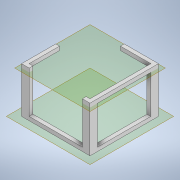
# Autodesk Inventor part: mousecap
Saved by Autodesk Inventor 2022 (Build 260153000, 153)
## iProperties
Created: 2022-02-16
Part Number: mousecap
Material: Generic
Document SubType Name: Modeling
Designer: Cornell
Density: 1 g/cm^3
Appearance: Default
Author: Cornell
Autodesk Inventor part; units mm, degrees
ref_plane "YZ Plane" through (0, 0, 0) normal (1, 0, 0) x (0, 1, 0)
ref_plane "XZ Plane" through (0, 0, 0) normal (0, 1, 0) x (-1, 0, 0)
ref_plane "XY Plane" through (0, 0, 0) normal (0, 0, 1) x (1, 0, 0)
sketch "Sketch1" plane through (0, 0, 0) normal (0, 1, 0) x (-1, 0, 0)
  line L0 (-9, -9) -> (-9, 9)
  line L1 (-9, 9) -> (9, 9)
  line L2 (-8, -8) -> (-8, 8)
  line L3 (-8, 8) -> (8, 8)
  line L4 (0, -8) -> (0, -9)
  line L5 (0, -9) -> (-1, -9)
  line L6 (-8, -8) -> (0, -8)
  line L7 (-9, -9) -> (0, -9)
  line L8 (9, 0) -> (9, 9)
  line L9 (8, 8) -> (8, 1)
  line L10 (9, 0) -> (8, 0)
  line L11 (8, 0) -> (8, 1.1953)
  line L12 (8, 8) -> (8, 9)
  line L13 (-8, 8) -> (-8, 9)
  line L14 (9, 9) -> (8, 9)
  line L15 (-8, 9) -> (-9, 9)
  line L16 (8, 8) -> (7, 8)
  line L17 (7, 8) -> (7, 9)
  line L18 (-8, 8) -> (-7, 8)
  line L19 (-7, 9) -> (-8, 9)
  line L20 (-8, 8) -> (-7, 8)
  line L21 (-7, 8) -> (-7, 9)
  point P0 (0, 0)
  point P1 (0, 11.1675)
  dimension "d4" = 18
  dimension "d5" = 18
  dimension "d10" = 16
  dimension "d11" = 16
  dimension "d33" = 1
  dimension "d62" = 1
  dimension "d63" = 1
  constraints: 44 end point, 8 point on line, 5 perpendicular, 4 collinear, 2 horizontal, 1 vertical
  measures "d4" distance of L0.start L0.end
  measures "d5" distance of L0.end L1.end
  measures "d10" distance of L2.start L2.end
  measures "d11" distance of L2.end L3.end
  measures "d33" distance of L4.end L5.end
  measures "d62" distance of L3.end L16.end
  measures "d63" distance of L2.end L18.end
extrude "Extrusion1" add sketch "Sketch1" against normal blind 1 contours L0 L1 L13 L2 L6 L4 L5 L7 | L1 L21 L3 L13 | L1 L12 L3 L17 | L1 L8 L10 L11 L9 L12
ref_plane "Work Plane1" through (0, -12, 0) normal (0, -1, 0) x (1, 0, 0)
ref_plane "Work Plane6" through (0, -1, 0) normal (0, -1, 0) x (1, 0, 0)
sketch "Sketch11" plane through (0, -1, 0) normal (0, -1, 0) x (1, 0, 0)
  line L0 (9, 9) -> (-9, 9) projected
  line L1 (-9, 9) -> (-9, 7)
  line L2 (-9, 0) -> (-9, 9) projected
  line L3 (-8, 0) -> (-8, 8) projected
  line L4 (-8, 8) -> (8, 8) projected
  line L5 (-8, 7) -> (-8, 8)
  line L6 (-8, 8) -> (-7, 8)
  line L7 (-7, 8) -> (-7, 9)
  line L8 (-7, 9) -> (-9, 9)
  line L9 (-9, 7) -> (-8, 7)
  line L10 (9, -9) -> (9, 9) projected
  line L11 (9, 9) -> (7, 9)
  line L12 (7, 9) -> (7, 8)
  line L13 (7, 8) -> (8, 8)
  line L14 (8, 8) -> (8, 7)
  line L15 (8, 8) -> (8, -8) projected
  line L16 (9, 7) -> (9, 9)
  line L17 (8, 7) -> (9, 7)
  line L18 (8, -7.9765) -> (8, -6.9765)
  line L19 (8, -6.9765) -> (9, -6.9765)
  line L20 (9, -9) -> (7, -9)
  line L21 (0, -9) -> (9, -9) projected
  line L22 (8, -8) -> (0, -8) projected
  line L23 (7, -8) -> (8, -8)
  line L24 (8, -8) -> (7, -8)
  line L25 (7, -9) -> (7, -8)
  point P0 (0, 0)
  dimension "d54" = 2
  dimension "d55" = 1
  dimension "d56" = 2
  dimension "d57" = 1
  constraints: 36 end point, 14 point on line, 8 perpendicular, 2 collinear, 1 parallel
  measures "d54" distance of L0.end L1.end
  measures "d55" distance of L3.end L6.end
  measures "d56" distance of L0.start L11.end
  measures "d57" distance of L18.start L18.end
extrude "Extrusion5" add sketch "Sketch11" along normal blind 10 contours L10 L17 L14 L4 L12 L0 | L7 L4 L3 L9 L1 L0 | L10 L20 L25 L22 L15 L19
sketch "Sketch12" plane through (0, -12, 0) normal (0, -1, 0) x (1, 0, 0)
  line L0 (9, 9) -> (9, -9) projected
  line L1 (9, 9) -> (9, -9)
  line L2 (9, -9) -> (7.0041, -9)
  line L3 (9, -9) -> (0, -9) projected
  line L4 (7, -8) -> (7, -9) projected
  line L5 (7, -8) -> (8, -8)
  line L6 (8, -8) -> (8, 8) projected
  line L7 (8, -8) -> (8, 8)
  line L8 (8, 8) -> (-8, 8) projected
  line L9 (8, 8) -> (-8, 8)
  line L10 (-8, 8) -> (-8, 7.0773)
  line L11 (-8, 8) -> (-8, 0) projected
  line L12 (-8, 7) -> (-9, 7) projected
  line L13 (-9, 0) -> (-9, 9) projected
  line L14 (-9, 7) -> (-9, 9)
  line L15 (-9, 9) -> (9, 9) projected
  line L16 (-9, 9) -> (9, 9)
  point P0 (0, 0)
  constraints: 16 end point, 3 collinear, 2 point on line, 1 horizontal, 1 perpendicular, 1 vertical
extrude "Extrusion6" add sketch "Sketch12" against normal blind 1
body "Solid1"
